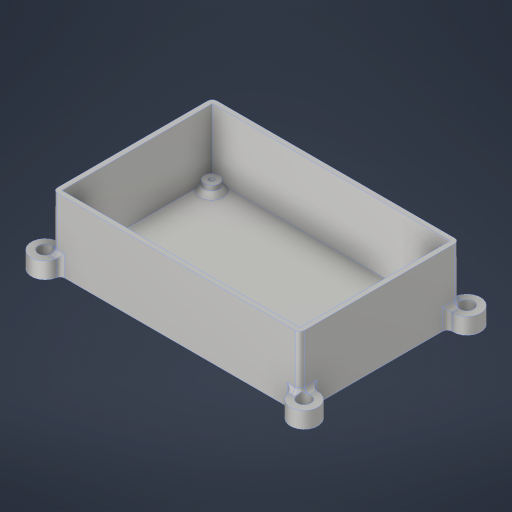
# Autodesk Inventor part: Orange Pi Case
Saved by Autodesk Inventor 2023 (Build 270158000, 158)
## iProperties
Created: 2024-02-12
Part Number: Orange Pi Case
Material: Aluminum 6061
Document SubType Name: Modeling
Designer: dlangdon
Density: 2.7 g/cm^3
Appearance: Aluminum - Flat
Author: dlangdon
Autodesk Inventor part; units mm, degrees
ref_plane "YZ Plane" through (0, 0, 0) normal (1, 0, 0) x (0, 1, 0)
ref_plane "XZ Plane" through (0, 0, 0) normal (0, 1, 0) x (-1, 0, 0)
ref_plane "XY Plane" through (0, 0, 0) normal (0, 0, 1) x (1, 0, 0)
sketch "Sketch1" plane through (0, 0, 0) normal (0, 1, 0) x (-1, 0, 0)
  line L0 (46.9275, 27.945) -> (-46.9275, 27.945) construction
  line L1 (-46.9275, 27.945) -> (-46.9275, -27.945) construction
  line L2 (-46.9275, -27.945) -> (46.9275, -27.945) construction
  line L3 (46.9275, -27.945) -> (46.9275, 27.945) construction
  line L4 (46.9275, 27.945) -> (-46.9275, -27.945) construction
  line L5 (-46.9275, 27.945) -> (46.9275, -27.945) construction
  line L6 (51, 32.25) -> (-51, 32.25) construction
  line L7 (-51, 32.25) -> (-51, -32.25) construction
  line L8 (-51, -32.25) -> (51, -32.25) construction
  line L9 (51, -32.25) -> (51, 32.25) construction
  line L10 (51, 32.25) -> (-51, -32.25) construction
  line L11 (-51, 32.25) -> (51, -32.25) construction
  line L12 (-53, 34.25) -> (53, 34.25)
  line L13 (53, 34.25) -> (53, -34.25)
  line L14 (53, -34.25) -> (-53, -34.25)
  line L15 (-53, -34.25) -> (-53, 34.25)
  line L16 (-53, 34.25) -> (53, -34.25) construction
  line L17 (53, 34.25) -> (-53, -34.25) construction
  point P0 (0, 0)
  dimension "d0" = 55.89
  dimension "d1" = 93.855
  dimension "d2" = 102
  dimension "d3" = 64.5
  dimension "d4" = 2
  dimension "d5" = 2
  constraints: 36 end point, 6 midpoint, 6 parallel, 4 coincident, 3 horizontal, 3 perpendicular
  measures "d0" distance of L2.end L0.start
  measures "d1" distance of L0.start L0.end
  measures "d2" distance of L8.end L7.end
  measures "d3" distance of L6.end L7.end
  measures "d4" distance between parallel lines of L9 L13
  measures "d5" distance between parallel lines of L8 L14
extrude "Extrusion1" add sketch "Sketch1" along normal blind 30
fillet "Fillet1" radius 2 4 edges at (53, 15, 34.25) (53, 15, -34.25) (-53, 15, -34.25) (-53, 15, 34.25)
shell "Shell1" thickness 2 removed faces 1 at (-17, 30, -11.4167)
hole "Hole1" at (46.9275, 0, 27.945) at (46.9275, 0, -27.945) at (-46.9275, 0, -27.945) at (-46.9275, 0, 27.945) direction (0, 1, 0) diameter 2.459 end through all thread size "M3x0.5" class "6H" standard "ISO Metric profile"
sketch "Sketch2" plane through (-51, 2, -32.25) normal (0, 1, 0) x (1, 0, 0)
  circle A0 centre (4.0725, -4.305) radius 1.2295 projected
  circle A1 centre (97.9275, -60.195) radius 1.2295 projected
  circle A2 centre (97.9275, -4.305) radius 1.2295 projected
  circle A3 centre (4.0725, -60.195) radius 1.2295 projected
  line L0 (102, -64.5) -> (102, 0) projected
  line L1 (102, 0) -> (0, 0) projected
  line L2 (0, 0) -> (0, -64.5) projected
  line L3 (0, -64.5) -> (102, -64.5) projected
  circle A4 centre (4.0725, -60.195) radius 3.2295
  circle A5 centre (4.0725, -4.305) radius 3.2295
  circle A6 centre (97.9275, -4.305) radius 3.2295
  circle A7 centre (97.9275, -60.195) radius 3.2295
  point P0 (51, -32.25)
  dimension "d17" = 2
  constraints: 4 centre point, 3 equal radius
  measures "d17" radial gap between concentric circles of A3 A4
extrude "Extrusion2" add sketch "Sketch2" along normal blind 4 contours A4 | A5 | A6 | A7
chamfer "Chamfer1" distance 2 angle 45 4 edges at (-50.157, 2, -27.945) (-50.157, 2, 27.945) (43.698, 2, 27.945) (43.698, 2, -27.945)
sketch "Sketch3" plane through (0, 0, 0) normal (0, -1, 0) x (1, 0, 0)
  line L0 (55.5625, 34.925) -> (-55.5625, 34.925) construction
  line L1 (-55.5625, 34.925) -> (-55.5625, -34.925) construction
  line L2 (-55.5625, -34.925) -> (55.5625, -34.925) construction
  line L3 (55.5625, -34.925) -> (55.5625, 34.925) construction
  line L4 (55.5625, 34.925) -> (-55.5625, -34.925) construction
  line L5 (-55.5625, 34.925) -> (55.5625, -34.925) construction
  circle A0 centre (-55.5625, 34.925) radius 2.9
  circle A1 centre (-55.5625, 34.925) radius 5.9
  circle A2 centre (-55.5625, -34.925) radius 5.9
  circle A3 centre (-55.5625, -34.925) radius 2.9
  circle A4 centre (55.5625, -34.925) radius 5.9
  circle A5 centre (55.5625, -34.925) radius 2.9
  circle A6 centre (55.5625, 34.925) radius 5.9
  circle A7 centre (55.5625, 34.925) radius 2.9
  line L6 (51, -32.25) -> (51, 32.25) projected
  line L7 (51, 32.25) -> (-51, 32.25) projected
  line L8 (-51, 32.25) -> (-51, -32.25) projected
  line L9 (-51, -32.25) -> (51, -32.25) projected
  arc A8 (-51, 34.25) -> (-53, 32.25) centre (-51, 32.25) ccw projected
  line L10 (-51, 34.25) -> (51, 34.25) projected
  arc A9 (53, 32.25) -> (51, 34.25) centre (51, 32.25) ccw projected
  line L11 (53, 32.25) -> (53, -32.25) projected
  arc A10 (51, -34.25) -> (53, -32.25) centre (51, -32.25) ccw projected
  line L12 (51, -34.25) -> (-51, -34.25) projected
  arc A11 (-53, -32.25) -> (-51, -34.25) centre (-51, -32.25) ccw projected
  line L13 (-53, -32.25) -> (-53, 32.25) projected
  point P0 (0, 0)
  point P1 (51, -31.1842)
  point P2 (50.3038, -32.25)
  point P3 (50.3038, 32.25)
  point P4 (51, 31.1842)
  point P5 (-51, 31.1842)
  point P6 (-50.3038, 32.25)
  point P7 (-50.3038, -32.25)
  point P8 (-51, -31.1842)
  dimension "d23" = 111.125
  dimension "d24" = 69.85
  dimension "d25" = 5.8
  dimension "d26" = 3
  constraints: 12 end point, 8 centre point, 7 coincident, 6 equal radius, 2 midpoint, 2 parallel, 1 horizontal, 1 perpendicular
  measures "d23" distance of L1.end L2.end
  measures "d24" distance of L0.end L1.end
  measures "d25" diameter of A0
  measures "d26" radial gap between concentric circles of A1 A0
extrude "Extrusion3" add sketch "Sketch3" against normal blind 7 contours A1 L10 A8 L13 | L13 A8 L10 A1 L7 L8 | L13 A11 L12 A2 | A2 L8 L9 L12 A11 L13 | L10 A9 L11 A6 L6 L7 | A6 L11 A9 L10 | L9 L6 A4 L11 A10 L12 | L12 A10 L11 A4
fillet "Fillet2" radius 2 12 edges at (-49.7012, 3.5, 34.25) (-50.3506, 7, 34.25) (50.3506, 7, 34.25) (49.7012, 3.5, 34.25) (49.7012, 3.5, -34.25) (50.3506, 7, -34.25) (-50.3506, 7, -34.25) (-49.7012, 3.5, -34.25) (-53, 3.5, -29.6105) (-53, 3.5, 29.6105) (53, 3.5, -29.6105) (53, 3.5, 29.6105)
body "Solid1"
